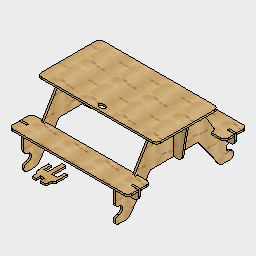
Picnic Table To Go Assembly v11 (Autodesk Fusion 360 design; units mm, degrees)
Autodesk Fusion 360 part; units mm, degrees
note: some values were not read from the file. Set by a fixed rule: which sketch regions a step uses.
sketch "Sketch1" plane through (0, 0, 0) normal (1, 0, 0) x (0, 1, 0) in component "Table Leg 1"
  line L0 (0, 0) -> (0, 304.8)
  line L1 (0, 304.8) -> (101.6, 304.8)
  line L2 (101.6, 304.8) -> (101.6, 234.95)
  line L3 (101.6, 234.95) -> (120.6183, 234.95)
  line L4 (120.6183, 234.95) -> (120.6183, 304.8)
  line L5 (120.6183, 304.8) -> (222.25, 304.8)
  line L6 (222.25, 304.8) -> (222.25, 323.8182)
  line L7 (222.25, 323.8182) -> (184.15, 323.8182)
  line L8 (184.15, 323.8182) -> (355.6, 609.6)
  line L9 (355.6, 609.6) -> (812.8, 609.6)
  line L10 (812.8, 609.6) -> (984.25, 323.8182)
  line L11 (984.25, 323.8182) -> (946.15, 323.8182)
  line L12 (946.15, 323.8182) -> (946.15, 304.8)
  line L13 (946.15, 304.8) -> (1047.7818, 304.8)
  line L14 (1047.7818, 304.8) -> (1047.7817, 234.95)
  line L15 (1047.7818, 234.95) -> (1066.8, 234.95)
  line L16 (1066.8, 234.95) -> (1066.8, 304.8)
  line L17 (1066.8, 304.8) -> (1168.4, 304.8)
  line L18 (1168.4, 304.8) -> (1168.4, 0)
  line L19 (1168.4, 0) -> (1034.5613, 0)
  line L20 (1034.5613, 0) -> (819.15, 304.8)
  line L21 (819.15, 304.8) -> (349.25, 304.8)
  line L22 (349.25, 304.8) -> (133.8387, 0)
  line L23 (133.8387, 0) -> (0, 0)
  line L24 (584.2, 304.8) -> (584.2, 609.6) construction
  line L25 (574.6909, 609.6) -> (574.6909, 635)
  line L26 (574.6909, 635) -> (574.6909, 493.776)
  line L27 (574.6909, 493.776) -> (593.7091, 493.776)
  line L28 (593.7091, 493.776) -> (593.7091, 609.6)
  circle A0 centre (482.6, 558.8) radius 50.8
  line L29 (431.8, 558.8) -> (533.4, 558.8)
  circle A1 centre (685.8, 558.8) radius 50.8
  line L30 (635, 558.8) -> (736.6, 558.8)
  arc A2 (114.1106, 0) -> (145.2246, 16.1108) centre (114.1106, 38.1) ccw
  arc A3 (38.1, 76.2) -> (38.1, 0) centre (38.1, 38.1) ccw
  arc A4 (0, 190.5) -> (38.1, 152.4) centre (38.1, 190.5) ccw
  arc A5 (38.1, 76.2) -> (38.1, 152.4) centre (38.1, 114.3) ccw
  arc A6 (368.9781, 304.8) -> (337.864, 288.6892) centre (368.9781, 266.7) ccw
  arc A7 (830.536, 288.6892) -> (799.4219, 304.8) centre (799.4219, 266.7) ccw
  arc A8 (1023.1754, 16.1108) -> (1054.2894, 0) centre (1054.2894, 38.1) ccw
  arc A9 (1130.3, 152.4) -> (1168.4, 190.5) centre (1130.3, 190.5) ccw
  arc A10 (1130.3, 152.4) -> (1130.3, 76.2) centre (1130.3, 114.3) ccw
  arc A11 (1130.3, 0) -> (1130.3, 76.2) centre (1130.3, 38.1) ccw
  arc A12 (823.8984, 591.1007) -> (791.2269, 609.6) centre (791.2269, 571.5) ccw
  arc A13 (377.1731, 609.6) -> (344.5016, 591.1007) centre (377.1731, 571.5) ccw
  arc A14 (195.6889, 343.0518) -> (206.5793, 323.8182) centre (206.5793, 336.5183) ccw
  arc A15 (961.8207, 323.8182) -> (972.7111, 343.0518) centre (961.8207, 336.5182) ccw
  line L31 (38.1, 114.3) -> (48.26, 114.3)
  line L32 (48.26, 114.3) -> (76.2, 114.3) construction
  line L33 (1130.3, 114.3) -> (1092.2, 114.3) construction
  dimension "d4" = 304.8
  dimension "d5" = 19.0183
  dimension "d6" = 38.1
  dimension "d7" = 19.0183
  dimension "d8" = 69.85
  dimension "d9" = 184.15
  dimension "d10" = 101.6
  dimension "d11" = 184.15
  dimension "d12" = 254
  dimension "d13" = 469.9
  dimension "d14" = 1168.4
  dimension "d15" = 304.8
  dimension "d16" = 374.65
  dimension "d17" = 115.824
  dimension "d18" = 19.0183
  dimension "d19" = 101.6
  dimension "d20" = 101.6
  dimension "d21" = 101.6
  dimension "d23" = 38.1
  dimension "d24" = 38.1
  dimension "d25" = 38.1
  dimension "d26" = 76.2
  dimension "d27" = 38.1
  dimension "d28" = 38.1
  dimension "d29" = 38.1
  dimension "d30" = 38.1
  dimension "d31" = 38.1
  dimension "d32" = 38.1
  dimension "d33" = 38.1
  dimension "d34" = 76.2
  dimension "d35" = 12.7
  dimension "d36" = 12.7
  dimension "d37" = 38.1
  dimension "d38" = 38.1
  dimension "d200" = 225.425
  dimension "d230" = 0
  dimension "d231" = 0
  dimension "d232" = 0
  dimension "d233" = 0
  dimension "d270" = 0
  dimension "d271" = 0
  dimension "d272" = 0
  dimension "d273" = 0
  dimension "d495" = 0
  dimension "d496" = 0
  dimension "d497" = 0
  dimension "d498" = 0
  dimension "d543" = 457.2
  dimension "d545" = 70.48
  dimension "d556" = 0
  dimension "d557" = 0
  dimension "d558" = 0
  dimension "d559" = 0
  dimension "d564" = 70.5
  dimension "d566" = 0
  dimension "d567" = 0
  dimension "d568" = 0
  dimension "d569" = 0
  dimension "d601" = 609.6
  dimension "d602" = 311.15
  dimension "d604" = 0
  dimension "d605" = 0
  dimension "d606" = 0
  dimension "d607" = 0
  dimension "d636" = 0
  dimension "d637" = 0
  dimension "d638" = 0
  dimension "d639" = 0
  dimension "d652" = 0
  dimension "d653" = 0
  dimension "d654" = 0
  dimension "d655" = 0
  measures "d4" distance of L0.start L0.end
  measures "d5" distance of L5.end L6.end
  measures "d6" distance of L6.end L7.end
  measures "d7" distance of L2.end L3.end
  measures "d8" distance of L3.end L4.end
  measures "d10" distance of L0.end L1.end
  measures "d11" distance of L0 L7.end
  measures "d13" distance of L20.end L21.end
  measures "d14" distance of L0 L18
  measures "d15" distance of L9 L21
  measures "d17" distance of L27.end L28.end
  measures "d18" distance of L26.end L27.end
  measures "d19" distance of L24 A0.centre
  measures "d20" diameter of A0
  measures "d21" distance of L24 A1.centre
  measures "d23" radius of A3
  measures "d24" radius of A5
  measures "d25" radius of A4
  measures "d26" distance of L0 L32.end
  measures "d27" radius of A2
  measures "d28" radius of A6
  measures "d29" radius of A7
  measures "d30" radius of A8
  measures "d31" radius of A11
  measures "d32" radius of A10
  measures "d33" radius of A9
  measures "d34" distance of L18 L33.end
  measures "d35" radius of A14
  measures "d36" radius of A15
  measures "d37" radius of A12
  measures "d38" radius of A13
  measures "d543" distance of L8.end L9.end
  measures "d564" angle of L20 L22
  measures "d601" distance of L8.end L23
extrude "Extrude1" add sketch "Sketch1" along normal blind 18.2563 contours A1 L30 | A0 L29 | L0 L1 L2 L3 L4 L5 L6 L7 L8 L9 L10 L11 L12 L13 L14 L15 L16 L17 L18 L19 L20 L21 L22 L23 L26 L27 L28 A2 A3 A4 A5 A8 A9 A10 A11 A12 A13 A14 A15 picked at (681.0293, 575.0474) picked at (477.8293, 575.0474) makes body 1 in component "Table Leg 1"
sketch "Sketch1 (2)" plane through (0, 0, 0) normal (1, 0, 0) x (0, 1, 0) in component "Table Leg 2"
  line L0 (0, 0) -> (0, 304.8)
  line L1 (0, 304.8) -> (101.6, 304.8)
  line L2 (101.6, 304.8) -> (101.6, 234.95)
  line L3 (101.6, 234.95) -> (120.6183, 234.95)
  line L4 (120.6183, 234.95) -> (120.6183, 304.8)
  line L5 (120.6183, 304.8) -> (222.25, 304.8)
  line L6 (222.25, 304.8) -> (222.25, 323.8182)
  line L7 (222.25, 323.8182) -> (184.15, 323.8182)
  line L8 (184.15, 323.8182) -> (355.6, 609.6)
  line L9 (355.6, 609.6) -> (812.8, 609.6)
  line L10 (812.8, 609.6) -> (984.25, 323.8182)
  line L11 (984.25, 323.8182) -> (946.15, 323.8183)
  line L12 (946.15, 323.8183) -> (946.15, 304.8)
  line L13 (946.15, 304.8) -> (1047.7818, 304.8)
  line L14 (1047.7818, 304.8) -> (1047.7817, 234.95)
  line L15 (1047.7818, 234.95) -> (1066.8, 234.95)
  line L16 (1066.8, 234.95) -> (1066.8, 304.8)
  line L17 (1066.8, 304.8) -> (1168.4, 304.8)
  line L18 (1168.4, 304.8) -> (1168.4, 0)
  line L19 (1168.4, 0) -> (1034.5613, 0)
  line L20 (1034.5613, 0) -> (819.15, 304.8)
  line L21 (819.15, 304.8) -> (349.25, 304.8)
  line L22 (349.25, 304.8) -> (133.8387, 0)
  line L23 (133.8387, 0) -> (0, 0)
  line L24 (584.2, 304.8) -> (584.2, 609.6) construction
  line L25 (574.6909, 609.6) -> (574.6909, 635)
  line L26 (574.6909, 635) -> (574.6909, 493.776)
  line L27 (574.6909, 493.776) -> (593.7091, 493.776)
  line L28 (593.7091, 493.776) -> (593.7091, 609.6)
  circle A0 centre (482.6, 558.8) radius 50.8
  line L29 (431.8, 558.8) -> (533.4, 558.8)
  circle A1 centre (685.8, 558.8) radius 50.8
  line L30 (635, 558.8) -> (736.6, 558.8)
  arc A2 (114.1106, 0) -> (145.2246, 16.1108) centre (114.1106, 38.1) ccw
  arc A3 (38.1, 76.2) -> (38.1, 0) centre (38.1, 38.1) ccw
  arc A4 (0, 190.5) -> (38.1, 152.4) centre (38.1, 190.5) ccw
  arc A5 (38.1, 76.2) -> (38.1, 152.4) centre (38.1, 114.3) ccw
  arc A6 (368.9781, 304.8) -> (337.864, 288.6892) centre (368.9781, 266.7) ccw
  arc A7 (830.536, 288.6892) -> (799.4219, 304.8) centre (799.4219, 266.7) ccw
  arc A8 (1023.1754, 16.1108) -> (1054.2894, 0) centre (1054.2894, 38.1) ccw
  arc A9 (1130.3, 152.4) -> (1168.4, 190.5) centre (1130.3, 190.5) ccw
  arc A10 (1130.3, 152.4) -> (1130.3, 76.2) centre (1130.3, 114.3) ccw
  arc A11 (1130.3, 0) -> (1130.3, 76.2) centre (1130.3, 38.1) ccw
  arc A12 (823.8984, 591.1007) -> (791.2269, 609.6) centre (791.2269, 571.5) ccw
  arc A13 (377.1731, 609.6) -> (344.5016, 591.1007) centre (377.1731, 571.5) ccw
  arc A14 (195.6889, 343.0518) -> (206.5793, 323.8182) centre (206.5793, 336.5182) ccw
  arc A15 (961.8207, 323.8182) -> (972.7111, 343.0518) centre (961.8207, 336.5182) ccw
  line L31 (38.1, 114.3) -> (48.26, 114.3)
  line L32 (48.26, 114.3) -> (76.2, 114.3) construction
  line L33 (1130.3, 114.3) -> (1092.2, 114.3) construction
  dimension "d4_1" = 304.8
  dimension "d5_1" = 19.0183
  dimension "d6_1" = 38.1
  dimension "d7_1" = 19.0183
  dimension "d8_1" = 69.85
  dimension "d9_1" = 184.15
  dimension "d10_1" = 101.6
  dimension "d11_1" = 184.15
  dimension "d12_1" = 254
  dimension "d13_1" = 469.9
  dimension "d14_1" = 1168.4
  dimension "d15_1" = 304.8
  dimension "d16_1" = 374.65
  dimension "d17_1" = 115.824
  dimension "d18_1" = 19.0183
  dimension "d19_1" = 101.6
  dimension "d20_1" = 101.6
  dimension "d21_1" = 101.6
  dimension "d23_1" = 38.1
  dimension "d24_1" = 38.1
  dimension "d25_1" = 38.1
  dimension "d26_1" = 76.2
  dimension "d27_1" = 38.1
  dimension "d28_1" = 38.1
  dimension "d29_1" = 38.1
  dimension "d30_1" = 38.1
  dimension "d31_1" = 38.1
  dimension "d32_1" = 38.1
  dimension "d33_1" = 38.1
  dimension "d34_1" = 76.2
  dimension "d35_1" = 12.7
  dimension "d36_1" = 12.7
  dimension "d37_1" = 38.1
  dimension "d38_1" = 38.1
  dimension "d218" = 0
  dimension "d219" = 0
  dimension "d220" = 0
  dimension "d221" = 0
  dimension "d254" = 0
  dimension "d255" = 0
  dimension "d256" = 0
  dimension "d257" = 0
  dimension "d262" = 0
  dimension "d263" = 0
  dimension "d264" = 0
  dimension "d265" = 0
  dimension "d471" = 0
  dimension "d472" = 0
  dimension "d473" = 0
  dimension "d474" = 0
  dimension "d487" = 0
  dimension "d488" = 0
  dimension "d489" = 0
  dimension "d490" = 0
  dimension "d544" = 457.2
  dimension "d548" = 0
  dimension "d549" = 0
  dimension "d550" = 0
  dimension "d551" = 0
  dimension "d565" = 70.5
  dimension "d603" = 609.6
  dimension "d628" = 0
  dimension "d629" = 0
  dimension "d630" = 0
  dimension "d631" = 0
  measures "d4_1" distance of L0.start L0.end
  measures "d5_1" distance of L5.end L6.end
  measures "d6_1" distance of L6.end L7.end
  measures "d7_1" distance of L2.end L3.end
  measures "d8_1" distance of L3.end L4.end
  measures "d10_1" distance of L0.end L1.end
  measures "d11_1" distance of L0 L7.end
  measures "d13_1" distance of L20.end L21.end
  measures "d14_1" distance of L0 L18
  measures "d15_1" distance of L9 L21
  measures "d17_1" distance of L27.end L28.end
  measures "d18_1" distance of L26.end L27.end
  measures "d19_1" distance of L24 A0.centre
  measures "d20_1" diameter of A0
  measures "d21_1" distance of L24 A1.centre
  measures "d23_1" radius of A3
  measures "d24_1" radius of A5
  measures "d25_1" radius of A4
  measures "d26_1" distance of L0 L32.end
  measures "d27_1" radius of A2
  measures "d28_1" radius of A6
  measures "d29_1" radius of A7
  measures "d30_1" radius of A8
  measures "d31_1" radius of A11
  measures "d32_1" radius of A10
  measures "d33_1" radius of A9
  measures "d34_1" distance of L18 L33.end
  measures "d35_1" radius of A14
  measures "d36_1" radius of A15
  measures "d37_1" radius of A12
  measures "d38_1" radius of A13
  measures "d544" distance of L8.end L9.end
  measures "d565" angle of L20 L22
  measures "d603" distance of L8.end L23
extrude "Extrude1'" add sketch "Sketch1 (2)" along normal blind 18.2563 separate body contours A1 L30 | A0 L29 | L0 L1 L2 L3 L4 L5 L6 L7 L8 L9 L10 L11 L12 L13 L14 L15 L16 L17 L18 L19 L20 L21 L22 L23 L26 L27 L28 A2 A3 A4 A5 A8 A9 A10 A11 A12 A13 A14 A15 picked at (690.3983, 577.4573) picked at (480.1901, 575.561) makes body 2 in component "Table Leg 2"
sketch "Sketch1 (3)" plane through (0, 0, 0) normal (0, 1, 0) x (1, 0, 0) in component "Tabletop Support"
  line L0 (-50.8, -304.8) -> (1117.6, -304.8)
  line L1 (1117.6, -304.8) -> (1066.8, 0)
  line L2 (1066.8, 0) -> (990.6, 0)
  line L3 (990.6, 0) -> (990.6, -188.976)
  line L4 (990.6, -188.976) -> (971.5818, -188.976)
  line L5 (971.5818, -188.976) -> (971.5818, 0)
  line L6 (971.5818, 0) -> (887.6566, 0)
  line L7 (887.6566, 0) -> (762, -177.8)
  line L8 (762, -177.8) -> (304.8, -177.8)
  line L9 (304.8, -177.8) -> (179.1434, 0)
  line L10 (179.1434, 0) -> (95.2182, 0)
  line L11 (95.2182, 0) -> (95.2183, -188.976)
  line L12 (95.2183, -188.976) -> (76.2, -188.976)
  line L13 (76.2, -188.976) -> (76.2, 0)
  line L14 (76.2, 0) -> (0, 0)
  line L15 (0, 0) -> (-50.8, -304.8)
  line L16 (533.4, -177.8) -> (533.4, -304.8) construction
  arc A0 (1072.1061, -31.8364) -> (1034.5245, 0) centre (1034.5245, -38.1) ccw
  arc A1 (907.3847, 0) -> (876.2707, -16.1108) centre (907.3847, -38.1) ccw
  arc A2 (190.5293, -16.1108) -> (159.4153, 0) centre (159.4153, -38.1) ccw
  arc A3 (32.2755, 0) -> (-5.3061, -31.8364) centre (32.2755, -38.1) ccw
  dimension "d41" = 355.6
  dimension "d42" = 19.0183
  dimension "d43" = 50.8
  dimension "d44" = 76.2
  dimension "d45" = 184.15
  dimension "d46" = 115.824
  dimension "d48" = 127
  dimension "d49" = 457.2
  dimension "d50" = 374.65
  dimension "d51" = 38.1
  dimension "d52" = 38.1
  dimension "d53" = 38.1
  dimension "d54" = 38.1
  dimension "d201" = 188.976
  dimension "d242" = 0
  dimension "d243" = 0
  dimension "d244" = 0
  dimension "d245" = 0
  dimension "d455" = 0
  dimension "d456" = 0
  dimension "d457" = 0
  dimension "d458" = 0
  dimension "d463" = 0
  dimension "d464" = 0
  dimension "d465" = 0
  dimension "d466" = 0
  dimension "d479" = 0
  dimension "d480" = 0
  dimension "d481" = 0
  dimension "d482" = 0
  dimension "d546" = 70.5
  dimension "d547" = 1168.4
  measures "d42" distance of L11.end L12.end
  measures "d43" distance of L0.start L14.end
  measures "d44" distance of L13.end L14.end
  measures "d46" distance of L0 L12
  measures "d48" distance of L0 L8
  measures "d49" distance of L7.end L8.end
  measures "d51" radius of A3
  measures "d52" radius of A2
  measures "d53" radius of A1
  measures "d54" radius of A0
  measures "d201" distance of L12 L14
  measures "d546" angle of L7 L9
  measures "d547" distance of L0.start L0.end
extrude "Extrude1''" add sketch "Sketch1 (3)" along normal blind 18.2563 separate body contours L0 L1 L2 L3 L4 L5 L6 L7 L8 L9 L10 L11 L12 L13 L14 L15 A0 A1 A2 A3 makes body 3 in component "Tabletop Support"
sketch "Sketch1 (4)" plane through (0, 0, 0) normal (0, 0, 1) x (1, 0, 0) in component "Seat 1"
  line L0 (0, 0) -> (1168.4, 0)
  line L1 (1168.4, 0) -> (1168.4, 222.25)
  line L2 (1168.4, 222.25) -> (0, 222.25)
  line L3 (0, 222.25) -> (0, 0)
  line L4 (1168.4, 120.6341) -> (1098.55, 120.6341)
  line L5 (1098.55, 120.6341) -> (1098.55, 101.6159)
  line L6 (1098.55, 101.6159) -> (1168.4, 101.6159)
  line L7 (1168.4, 101.6159) -> (1168.4, 120.6341)
  line L8 (0, 120.6341) -> (69.85, 120.6341)
  line L9 (69.85, 120.6341) -> (69.85, 101.6159)
  line L10 (69.85, 101.6159) -> (0, 101.6159)
  line L11 (0, 101.6159) -> (0, 120.6341)
  line L12 (0, 111.125) -> (1168.4, 111.125) construction
  arc A0 (38.1, 222.25) -> (0, 184.15) centre (38.1, 184.15) ccw
  arc A1 (0, 38.1) -> (38.1, 0) centre (38.1, 38.1) ccw
  arc A2 (1130.3, 0) -> (1168.4, 38.1) centre (1130.3, 38.1) ccw
  arc A3 (1168.4, 184.15) -> (1130.3, 222.25) centre (1130.3, 184.15) ccw
  dimension "d81" = 1168.4
  dimension "d82" = 222.25
  dimension "d83" = 19.0183
  dimension "d84" = 69.85
  dimension "d85" = 38.1
  dimension "d86" = 38.1
  dimension "d87" = 38.1
  dimension "d88" = 38.1
  dimension "d314" = 0
  dimension "d315" = 0
  dimension "d316" = 0
  dimension "d317" = 0
  dimension "d446" = 0
  dimension "d447" = 0
  dimension "d448" = 0
  dimension "d449" = 0
  dimension "d684" = 0
  dimension "d685" = 0
  dimension "d686" = 0
  dimension "d687" = 0
  dimension "d725" = 0
  dimension "d726" = 0
  dimension "d727" = 0
  dimension "d728" = 0
  dimension "d733" = 0
  dimension "d734" = 0
  dimension "d735" = 0
  dimension "d736" = 0
  measures "d81" distance of L1.end L2.end
  measures "d82" distance of L0.end L1.end
  measures "d83" distance of L8.end L9.end
  measures "d84" distance of L8.start L8.end
  measures "d85" radius of A1
  measures "d86" radius of A0
  measures "d87" radius of A2
  measures "d88" radius of A3
extrude "Extrude1'''" add sketch "Sketch1 (4)" along normal blind 18.2563 separate body contours L0 L1 L2 L3 L4 L5 L6 L8 L9 L10 A0 A1 A2 A3 makes body 4 in component "Seat 1"
sketch "Sketch1 (5)" plane through (0, 0, 0) normal (0, 0, 1) x (1, 0, 0) in component "Seat 2"
  line L0 (0, 0) -> (1168.4, 0)
  line L1 (1168.4, 0) -> (1168.4, 222.25)
  line L2 (1168.4, 222.25) -> (0, 222.25)
  line L3 (0, 222.25) -> (0, 0)
  line L4 (1168.4, 120.6341) -> (1098.55, 120.6341)
  line L5 (1098.55, 120.6341) -> (1098.55, 101.6159)
  line L6 (1098.55, 101.6159) -> (1168.4, 101.6159)
  line L7 (1168.4, 101.6159) -> (1168.4, 120.6341)
  line L8 (0, 120.6341) -> (69.85, 120.6341)
  line L9 (69.85, 120.6341) -> (69.85, 101.6159)
  line L10 (69.85, 101.6159) -> (0, 101.6159)
  line L11 (0, 101.6159) -> (0, 120.6341)
  line L12 (0, 111.125) -> (1168.4, 111.125) construction
  arc A0 (38.1, 222.25) -> (0, 184.15) centre (38.1, 184.15) ccw
  arc A1 (0, 38.1) -> (38.1, 0) centre (38.1, 38.1) ccw
  arc A2 (1130.3, 0) -> (1168.4, 38.1) centre (1130.3, 38.1) ccw
  arc A3 (1168.4, 184.15) -> (1130.3, 222.25) centre (1130.3, 184.15) ccw
  dimension "d81_1" = 1168.4
  dimension "d82_1" = 222.25
  dimension "d83_1" = 19.0183
  dimension "d84_1" = 69.85
  dimension "d85_1" = 38.1
  dimension "d86_1" = 38.1
  dimension "d87_1" = 38.1
  dimension "d88_1" = 38.1
  dimension "d302" = 0
  dimension "d303" = 0
  dimension "d304" = 0
  dimension "d305" = 0
  dimension "d438" = 0
  dimension "d439" = 0
  dimension "d440" = 0
  dimension "d441" = 0
  dimension "d519" = 0
  dimension "d520" = 0
  dimension "d521" = 0
  dimension "d522" = 0
  dimension "d590" = 0
  dimension "d591" = 0
  dimension "d592" = 0
  dimension "d593" = 0
  dimension "d676" = 0
  dimension "d677" = 0
  dimension "d678" = 0
  dimension "d679" = 0
  dimension "d717" = 0
  dimension "d718" = 0
  dimension "d719" = 0
  dimension "d720" = 0
  measures "d81_1" distance of L1.end L2.end
  measures "d82_1" distance of L0.end L1.end
  measures "d83_1" distance of L8.end L9.end
  measures "d84_1" distance of L8.start L8.end
  measures "d85_1" radius of A1
  measures "d86_1" radius of A0
  measures "d87_1" radius of A2
  measures "d88_1" radius of A3
extrude "Extrude1''''" add sketch "Sketch1 (5)" along normal blind 18.2563 separate body contours L0 L1 L2 L3 L4 L5 L6 L8 L9 L10 A0 A1 A2 A3 makes body 5 in component "Seat 2"
sketch "Sketch1 (6)" plane through (0, 0, 0) normal (0, 1, 0) x (1, 0, 0) in component "Seat Support 1"
  line L0 (0, 0) -> (1168.4, 0)
  line L1 (1168.4, 0) -> (1168.4, -101.6)
  line L2 (1168.4, -101.6) -> (0, -101.6)
  line L3 (0, -101.6) -> (0, 0)
  line L4 (0, -50.8) -> (1168.4, -50.8) construction
  line L5 (69.85, -101.6) -> (1098.55, -101.6)
  line L6 (1098.55, -101.6) -> (1098.55, -82.5817)
  line L7 (1098.55, -82.5817) -> (69.85, -82.5817)
  line L8 (69.85, -82.5817) -> (69.85, -101.6)
  line L9 (584.2, 0) -> (584.2, -101.6) construction
  arc A0 (38.1, 0) -> (0, -38.1) centre (38.1, -38.1) ccw
  arc A1 (1168.4, -38.1) -> (1130.3, 0) centre (1130.3, -38.1) ccw
  line L10 (127, 0) -> (146.0182, 0)
  line L11 (146.0182, 0) -> (146.0182, -12.7)
  line L12 (146.0182, -12.7) -> (127, -12.7)
  line L13 (127, -12.7) -> (127, 0)
  line L14 (1022.3818, 0) -> (1041.4, 0)
  line L15 (1041.4, 0) -> (1041.4, -12.7)
  line L16 (1041.4, -12.7) -> (1022.3818, -12.7)
  line L17 (1022.3818, -12.7) -> (1022.3818, 0)
  dimension "d91" = 1168.4
  dimension "d92" = 101.6
  dimension "d93" = 19.0183
  dimension "d94" = 69.85
  dimension "d95" = 38.1
  dimension "d96" = 38.1
  dimension "d99" = 19.0183
  dimension "d100" = 127
  dimension "d198" = 69.8818
  dimension "d290" = 0
  dimension "d291" = 0
  dimension "d292" = 0
  dimension "d293" = 0
  dimension "d422" = 0
  dimension "d423" = 0
  dimension "d424" = 0
  dimension "d425" = 0
  dimension "d503" = 0
  dimension "d504" = 0
  dimension "d505" = 0
  dimension "d506" = 0
  dimension "d574" = 0
  dimension "d575" = 0
  dimension "d576" = 0
  dimension "d577" = 0
  dimension "d660" = 0
  dimension "d661" = 0
  dimension "d662" = 0
  dimension "d663" = 0
  dimension "d701" = 0
  dimension "d702" = 0
  dimension "d703" = 0
  dimension "d704" = 0
  measures "d91" distance of L1.end L2.end
  measures "d92" distance of L0.start L2.end
  measures "d93" distance of L5.start L7.end
  measures "d94" distance of L3 L8
  measures "d95" radius of A0
  measures "d96" radius of A1
  measures "d99" distance of L11.end L12.end
  measures "d100" distance of L3 L13
  measures "d198" distance of L7 L12
extrude "Extrude1'''''" add sketch "Sketch1 (6)" along normal blind 18.2563 separate body contours L0 L1 L2 L3 L6 L7 L8 A0 A1 L11 L12 L13 L15 L16 L17 makes body 6 in component "Seat Support 1"
sketch "Sketch1 (7)" plane through (0, 0, 0) normal (0, 1, 0) x (1, 0, 0) in component "Seat Support 2"
  line L0 (0, 0) -> (1168.4, 0)
  line L1 (1168.4, 0) -> (1168.4, -101.6)
  line L2 (1168.4, -101.6) -> (0, -101.6)
  line L3 (0, -101.6) -> (0, 0)
  line L4 (0, -50.8) -> (1168.4, -50.8) construction
  line L5 (69.85, -101.6) -> (1098.55, -101.6)
  line L6 (1098.55, -101.6) -> (1098.55, -82.5817)
  line L7 (1098.55, -82.5817) -> (69.85, -82.5817)
  line L8 (69.85, -82.5817) -> (69.85, -101.6)
  line L9 (584.2, 0) -> (584.2, -101.6) construction
  arc A0 (38.1, 0) -> (0, -38.1) centre (38.1, -38.1) ccw
  arc A1 (1168.4, -38.1) -> (1130.3, 0) centre (1130.3, -38.1) ccw
  line L10 (127, 0) -> (146.0182, 0)
  line L11 (146.0182, 0) -> (146.0182, -12.7)
  line L12 (146.0182, -12.7) -> (127, -12.7)
  line L13 (127, -12.7) -> (127, 0)
  line L14 (1022.3818, 0) -> (1041.4, 0)
  line L15 (1041.4, 0) -> (1041.4, -12.7)
  line L16 (1041.4, -12.7) -> (1022.3818, -12.7)
  line L17 (1022.3818, -12.7) -> (1022.3818, 0)
  dimension "d91_1" = 1168.4
  dimension "d92_1" = 101.6
  dimension "d93_1" = 19.0183
  dimension "d94_1" = 69.85
  dimension "d95_1" = 38.1
  dimension "d96_1" = 38.1
  dimension "d99_1" = 19.0183
  dimension "d100_1" = 127
  dimension "d199" = 69.8818
  dimension "d278" = 0
  dimension "d279" = 0
  dimension "d280" = 0
  dimension "d281" = 0
  dimension "d430" = 0
  dimension "d431" = 0
  dimension "d432" = 0
  dimension "d433" = 0
  dimension "d511" = 0
  dimension "d512" = 0
  dimension "d513" = 0
  dimension "d514" = 0
  dimension "d582" = 0
  dimension "d583" = 0
  dimension "d584" = 0
  dimension "d585" = 0
  dimension "d668" = 0
  dimension "d669" = 0
  dimension "d670" = 0
  dimension "d671" = 0
  dimension "d709" = 0
  dimension "d710" = 0
  dimension "d711" = 0
  dimension "d712" = 0
  measures "d91_1" distance of L1.end L2.end
  measures "d92_1" distance of L0.start L2.end
  measures "d93_1" distance of L5.start L7.end
  measures "d94_1" distance of L3 L8
  measures "d95_1" radius of A0
  measures "d96_1" radius of A1
  measures "d99_1" distance of L11.end L12.end
  measures "d100_1" distance of L3 L13
  measures "d199" distance of L7 L12
extrude "Extrude1''''''" add sketch "Sketch1 (7)" along normal blind 18.2563 separate body contours L0 L1 L2 L3 L6 L7 L8 A0 A1 L11 L12 L13 L15 L16 L17 makes body 7 in component "Seat Support 2"
sketch "Sketch1 (8)" plane through (0, 0, 0) normal (0, 0, 1) x (1, 0, 0) in component "Tabletop"
  line L0 (0, 0) -> (1168.4, 0)
  line L1 (1168.4, 0) -> (1168.4, 609.6)
  line L2 (1168.4, 609.6) -> (0, 609.6)
  line L3 (0, 609.6) -> (0, 0)
  arc A0 (0, 38.1) -> (38.1, 0) centre (38.1, 38.1) ccw
  arc A1 (38.1, 609.6) -> (0, 571.5) centre (38.1, 571.5) ccw
  arc A2 (1168.4, 571.5) -> (1130.3, 609.6) centre (1130.3, 571.5) ccw
  arc A3 (1130.3, 0) -> (1168.4, 38.1) centre (1130.3, 38.1) ccw
  arc A4 (620.121, 50.8) -> (548.279, 50.8) centre (584.2, 38.1) ccw
  arc A5 (548.279, 50.8) -> (620.121, 50.8) centre (584.2, 63.5) ccw
  line L4 (584.2, 0) -> (584.2, 609.6) construction
  line L5 (584.2, 25.4) -> (584.2, 76.2) construction
  dimension "d150" = 38.1
  dimension "d151" = 38.1
  dimension "d152" = 38.1
  dimension "d153" = 38.1
  dimension "d154" = 609.6
  dimension "d155" = 1168.4
  dimension "d156" = 38.1
  dimension "d157" = 38.1
  dimension "d159" = 25.4
  dimension "d160" = 76.2
  dimension "d206" = 0
  dimension "d207" = 0
  dimension "d208" = 0
  dimension "d209" = 0
  measures "d150" radius of A0
  measures "d151" radius of A1
  measures "d152" radius of A3
  measures "d153" radius of A2
  measures "d154" distance of L0.start L2.end
  measures "d155" distance of L0.start L0.end
  measures "d156" radius of A5
  measures "d157" radius of A4
  measures "d159" distance of L0 L5.start
  measures "d160" distance of L0 L5.end
extrude "Extrude1'''''''" add sketch "Sketch1 (8)" along normal blind 18.2563 separate body contours L0 L1 L2 L3 A0 A1 A2 A3 makes body 8 in component "Tabletop"
sketch "Sketch2" plane through (0, 0, 0) normal (0, 0, -1) x (1, 0, 0) in component "Tabletop"
  arc A0 (620.121, -50.8) -> (548.279, -50.8) centre (584.2, -63.5) ccw
  arc A1 (548.279, -50.8) -> (620.121, -50.8) centre (584.2, -38.1) ccw
  arc A2 (1168.4, -38.1) -> (1130.3, 0) centre (1130.3, -38.1) ccw
  line L0 (1130.3, 0) -> (38.1, 0)
  arc A3 (38.1, 0) -> (0, -38.1) centre (38.1, -38.1) ccw
  line L1 (0, -38.1) -> (0, -571.5)
  arc A4 (0, -571.5) -> (38.1, -609.6) centre (38.1, -571.5) ccw
  line L2 (38.1, -609.6) -> (1130.3, -609.6)
  arc A5 (1130.3, -609.6) -> (1168.4, -571.5) centre (1130.3, -571.5) ccw
  line L3 (1168.4, -571.5) -> (1168.4, -38.1)
  line L4 (0, -304.8) -> (1168.4, -304.8) construction
  line L5 (145.6373, -295.2909) -> (444.0873, -295.2909)
  line L6 (444.0873, -295.2909) -> (444.0873, -230.7749)
  line L7 (444.0873, -230.7749) -> (145.6373, -230.7749)
  line L8 (145.6373, -230.7749) -> (145.6373, -295.2909)
  line L9 (145.6373, -314.3091) -> (444.0873, -314.3091)
  line L10 (444.0873, -314.3091) -> (444.0873, -378.8251)
  line L11 (444.0873, -378.8251) -> (145.6373, -378.8251)
  line L12 (145.6373, -378.8251) -> (145.6373, -314.3091)
  line L13 (1022.7628, -314.3091) -> (724.3128, -314.3091)
  line L14 (724.3128, -314.3091) -> (724.3128, -378.8251)
  line L15 (724.3128, -378.8251) -> (1022.7628, -378.8251)
  line L16 (1022.7628, -378.8251) -> (1022.7628, -314.3091)
  line L17 (1022.7628, -230.7749) -> (724.3128, -230.7749)
  line L18 (724.3128, -230.7749) -> (724.3128, -295.2909)
  line L19 (724.3128, -295.2909) -> (1022.7628, -295.2909)
  line L20 (1022.7628, -295.2909) -> (1022.7628, -230.7749)
  line L21 (444.0873, -295.2909) -> (444.0873, -314.3091) construction
  line L22 (724.3128, -295.2909) -> (724.3128, -314.3091) construction
  line L23 (145.6373, -295.2909) -> (145.6373, -97.7731)
  line L24 (1022.7628, -97.7731) -> (1022.7628, -295.2909)
  dimension "d163" = 19.0183
  dimension "d164" = 64.516
  dimension "d165" = 298.45
  measures "d163" distance of L5 L9
  measures "d164" distance of L5.start L7.end
  measures "d165" distance of L6.end L7.end
extrude "Extrude2" add sketch "Sketch2" along normal blind 18.2563 separate body contours L5 L6 L7 L8 L23 | L9 L10 L11 L12 | L13 L14 L15 L16 | L17 L18 L19 L20 L24 makes body 9 at (245.1206, 335.8145, 0) makes body 10 at (923.2794, 357.3198, 0) makes body 11 at (245.1206, 252.2802, 0) makes body 12 at (923.2794, 252.2802, 0) in component "Tabletop"
copy_body "Body->Comp1" bodies 9 removing the originals makes body 13 in component "Component"
copy_body "Body->Comp2" bodies 11 removing the originals makes body 14 in component "Component'"
copy_body "Body->Comp3" bodies 10 removing the originals makes body 15 in component "Component''"
copy_body "Body->Comp4" bodies 12 removing the originals makes body 16 in component "Component'''"
sketch "Sketch1 (9)" plane through (0, 0, 0) normal (0, 0, 1) x (1, 0, 0) in component "Carrying Clips"
  line L0 (25.4, 0) -> (63.5, 0)
  line L1 (63.5, 0) -> (63.5, 44.45)
  line L2 (63.5, 44.45) -> (101.6, 44.45)
  line L3 (101.6, 44.45) -> (101.6, 0)
  line L4 (101.6, 0) -> (158.75, 0)
  line L5 (184.15, 82.55) -> (184.15, 184.15)
  line L6 (184.15, 184.15) -> (158.75, 184.15)
  line L7 (158.75, 184.15) -> (158.75, 114.3)
  line L8 (158.75, 114.3) -> (101.6, 114.3)
  line L9 (101.6, 114.3) -> (101.6, 254)
  line L10 (101.6, 254) -> (63.5, 254)
  line L11 (63.5, 254) -> (63.5, 114.3)
  line L12 (63.5, 114.3) -> (25.4, 114.3)
  line L13 (25.4, 114.3) -> (25.4, 184.15)
  line L14 (25.4, 184.15) -> (0, 184.15)
  line L15 (0, 184.15) -> (0, 82.55)
  line L16 (0, 82.55) -> (0, 0) construction
  line L17 (0, 0) -> (25.4, 0) construction
  line L18 (25.4, 0) -> (25.4, 25.7539)
  arc A0 (0, 82.55) -> (12.7, 54.1519) centre (38.1, 82.55) ccw
  arc A1 (25.4, 25.7539) -> (12.7, 54.1519) centre (-12.7, 25.7539) ccw
  line L19 (158.75, 0) -> (158.75, 25.7539)
  arc A2 (171.45, 54.1519) -> (158.75, 25.7539) centre (196.85, 25.7539) ccw
  arc A3 (171.45, 54.1519) -> (184.15, 82.55) centre (146.05, 82.55) ccw
  line L20 (184.15, 82.55) -> (0, 82.55) construction
  dimension "d180" = 38.1
  dimension "d181" = 57.15
  dimension "d182" = 82.55
  dimension "d183" = 38.1
  dimension "d184" = 63.5
  dimension "d185" = 82.55
  dimension "d186" = 254
  dimension "d187" = 184.15
  dimension "d188" = 114.3
  dimension "d189" = 25.4
  dimension "d190" = 44.45
  dimension "d191" = 38.1
  dimension "d192" = 38.1
  dimension "d193" = 38.1
  dimension "d194" = 38.1
  dimension "d195" = 38.1
  dimension "d326" = 0
  dimension "d327" = 0
  dimension "d328" = 0
  dimension "d329" = 0
  dimension "d338" = 0
  dimension "d339" = 0
  dimension "d340" = 0
  dimension "d341" = 0
  dimension "d350" = 0
  dimension "d351" = 0
  dimension "d352" = 0
  dimension "d353" = 0
  dimension "d358" = 0
  dimension "d359" = 0
  dimension "d360" = 0
  dimension "d361" = 0
  dimension "d366" = 0
  dimension "d367" = 0
  dimension "d368" = 0
  dimension "d369" = 0
  dimension "d527" = 0
  dimension "d528" = 0
  dimension "d529" = 0
  dimension "d530" = 0
  dimension "d535" = 0
  dimension "d536" = 0
  dimension "d537" = 0
  dimension "d538" = 0
  dimension "d773" = 0
  dimension "d774" = 0
  dimension "d775" = 0
  dimension "d776" = 0
  dimension "d813" = 0
  dimension "d814" = 0
  dimension "d815" = 0
  dimension "d816" = 0
  measures "d180" distance of L11.end L12.end
  measures "d181" distance of L7.end L8.end
  measures "d182" distance of L3 L5
  measures "d183" distance of L1.end L2.end
  measures "d184" distance of L1 L15
  measures "d185" distance of L0 L15.end
  measures "d186" distance of L4 L10
  measures "d187" distance of L4 L6
  measures "d188" distance of L0 L12
  measures "d189" distance of L5.end L6.end
  measures "d190" distance of L2.end L3.end
  measures "d191" radius of A1
  measures "d192" radius of A0
  measures "d193" distance of L0.start L0.end
  measures "d194" radius of A2
  measures "d195" radius of A3
extrude "Extrude1''''''''" add sketch "Sketch1 (9)" along normal blind 18.2563 separate body makes body 17 in component "Carrying Clips"
sketch "Sketch1 (10)" plane through (0, 0, 0) normal (0, 0, 1) x (1, 0, 0) in component "Stock"
  line L0 (0, 0) -> (2438.4, 0)
  line L1 (2438.4, 0) -> (2438.4, 1219.2)
  line L2 (2438.4, 1219.2) -> (0, 1219.2)
  line L3 (0, 1219.2) -> (0, 0)
  dimension "d202" = 2438.4
  dimension "d203" = 1219.2
  dimension "d210" = 0
  dimension "d211" = 0
  dimension "d212" = 0
  dimension "d213" = 0
  dimension "d222" = 0
  dimension "d223" = 0
  dimension "d224" = 0
  dimension "d225" = 0
  dimension "d234" = 0
  dimension "d235" = 0
  dimension "d236" = 0
  dimension "d237" = 0
  dimension "d246" = 0
  dimension "d247" = 0
  dimension "d248" = 0
  dimension "d249" = 0
  dimension "d258" = 0
  dimension "d259" = 0
  dimension "d260" = 0
  dimension "d261" = 0
  dimension "d266" = 0
  dimension "d267" = 0
  dimension "d268" = 0
  dimension "d269" = 0
  dimension "d274" = 0
  dimension "d275" = 0
  dimension "d276" = 0
  dimension "d277" = 0
  dimension "d282" = 0
  dimension "d283" = 0
  dimension "d284" = 0
  dimension "d285" = 0
  dimension "d294" = 0
  dimension "d295" = 0
  dimension "d296" = 0
  dimension "d297" = 0
  dimension "d306" = 0
  dimension "d307" = 0
  dimension "d308" = 0
  dimension "d309" = 0
  dimension "d318" = 0
  dimension "d319" = 0
  dimension "d320" = 0
  dimension "d321" = 0
  dimension "d330" = 0
  dimension "d331" = 0
  dimension "d332" = 0
  dimension "d333" = 0
  dimension "d342" = 0
  dimension "d343" = 0
  dimension "d344" = 0
  dimension "d345" = 0
  dimension "d354" = 0
  dimension "d355" = 0
  dimension "d356" = 0
  dimension "d357" = 0
  dimension "d362" = 0
  dimension "d363" = 0
  dimension "d364" = 0
  dimension "d365" = 0
  dimension "d370" = 0
  dimension "d371" = 0
  dimension "d372" = 0
  dimension "d373" = 0
  dimension "d378" = 0
  dimension "d379" = 0
  dimension "d380" = 0
  dimension "d381" = 0
  dimension "d390" = 0
  dimension "d391" = 0
  dimension "d392" = 0
  dimension "d393" = 0
  dimension "d402" = 0
  dimension "d403" = 0
  dimension "d404" = 0
  dimension "d405" = 0
  dimension "d414" = 0
  dimension "d415" = 0
  dimension "d416" = 0
  dimension "d417" = 0
  dimension "d426" = 0
  dimension "d427" = 0
  dimension "d428" = 0
  dimension "d429" = 0
  dimension "d434" = 0
  dimension "d435" = 0
  dimension "d436" = 0
  dimension "d437" = 0
  dimension "d442" = 0
  dimension "d443" = 0
  dimension "d444" = 0
  dimension "d445" = 0
  dimension "d450" = 0
  dimension "d451" = 0
  dimension "d452" = 0
  dimension "d453" = 0
  dimension "d459" = 0
  dimension "d460" = 0
  dimension "d461" = 0
  dimension "d462" = 0
  dimension "d467" = 0
  dimension "d468" = 0
  dimension "d469" = 0
  dimension "d470" = 0
  dimension "d475" = 0
  dimension "d476" = 0
  dimension "d477" = 0
  dimension "d478" = 0
  dimension "d483" = 0
  dimension "d484" = 0
  dimension "d485" = 0
  dimension "d486" = 0
  dimension "d491" = 0
  dimension "d492" = 0
  dimension "d493" = 0
  dimension "d494" = 0
  dimension "d499" = 0
  dimension "d500" = 0
  dimension "d501" = 0
  dimension "d502" = 0
  dimension "d507" = 0
  dimension "d508" = 0
  dimension "d509" = 0
  dimension "d510" = 0
  dimension "d515" = 0
  dimension "d516" = 0
  dimension "d517" = 0
  dimension "d518" = 0
  dimension "d523" = 0
  dimension "d524" = 0
  dimension "d525" = 0
  dimension "d526" = 0
  dimension "d531" = 0
  dimension "d532" = 0
  dimension "d533" = 0
  dimension "d534" = 0
  dimension "d539" = 0
  dimension "d540" = 0
  dimension "d541" = 0
  dimension "d542" = 0
  dimension "d552" = 0
  dimension "d553" = 0
  dimension "d554" = 0
  dimension "d555" = 0
  dimension "d560" = 0
  dimension "d561" = 0
  dimension "d562" = 0
  dimension "d563" = 0
  dimension "d570" = 0
  dimension "d571" = 0
  dimension "d572" = 0
  dimension "d573" = 0
  dimension "d578" = 0
  dimension "d579" = 0
  dimension "d580" = 0
  dimension "d581" = 0
  dimension "d586" = 0
  dimension "d587" = 0
  dimension "d588" = 0
  dimension "d589" = 0
  dimension "d594" = 0
  dimension "d595" = 0
  dimension "d596" = 0
  dimension "d597" = 0
  dimension "d608" = 0
  dimension "d609" = 0
  dimension "d610" = 0
  dimension "d611" = 0
  dimension "d632" = 0
  dimension "d633" = 0
  dimension "d634" = 0
  dimension "d635" = 0
  dimension "d640" = 0
  dimension "d641" = 0
  dimension "d642" = 0
  dimension "d643" = 0
  dimension "d656" = 0
  dimension "d657" = 0
  dimension "d658" = 0
  dimension "d659" = 0
  dimension "d664" = 0
  dimension "d665" = 0
  dimension "d666" = 0
  dimension "d667" = 0
  dimension "d672" = 0
  dimension "d673" = 0
  dimension "d674" = 0
  dimension "d675" = 0
  dimension "d680" = 0
  dimension "d681" = 0
  dimension "d682" = 0
  dimension "d683" = 0
  dimension "d688" = 0
  dimension "d689" = 0
  dimension "d690" = 0
  dimension "d691" = 0
  dimension "d705" = 0
  dimension "d706" = 0
  dimension "d707" = 0
  dimension "d708" = 0
  dimension "d713" = 0
  dimension "d714" = 0
  dimension "d715" = 0
  dimension "d716" = 0
  dimension "d721" = 0
  dimension "d722" = 0
  dimension "d723" = 0
  dimension "d724" = 0
  dimension "d729" = 0
  dimension "d730" = 0
  dimension "d731" = 0
  dimension "d732" = 0
  dimension "d737" = 0
  dimension "d738" = 0
  dimension "d739" = 0
  dimension "d740" = 0
  dimension "d777" = 0
  dimension "d778" = 0
  dimension "d779" = 0
  dimension "d780" = 0
  dimension "d785" = 0
  dimension "d786" = 0
  dimension "d787" = 0
  dimension "d788" = 0
  dimension "d793" = 0
  dimension "d794" = 0
  dimension "d795" = 0
  dimension "d796" = 0
  dimension "d801" = 0
  dimension "d802" = 0
  dimension "d803" = 0
  dimension "d804" = 0
  dimension "d809" = 0
  dimension "d810" = 0
  dimension "d811" = 0
  dimension "d812" = 0
  dimension "d817" = 0
  dimension "d818" = 0
  dimension "d819" = 0
  dimension "d820" = 0
  dimension "d833" = 0
  dimension "d834" = 0
  dimension "d835" = 0
  dimension "d836" = 0
  dimension "d841" = 0
  dimension "d842" = 0
  dimension "d843" = 0
  dimension "d844" = 0
  dimension "d849" = 0
  dimension "d850" = 0
  dimension "d851" = 0
  dimension "d852" = 0
  dimension "d857" = 0
  dimension "d858" = 0
  dimension "d859" = 0
  dimension "d860" = 0
  measures "d202" distance of L0.start L0.end
  measures "d203" distance of L0.start L2.end
extrude "Extrude1'''''''''" add sketch "Sketch1 (10)" along normal blind 18.2563 separate body makes body 18 in component "Stock"
ref_plane "WorkPlane4" through (0, 0, 0) normal (0, 0, 1) x (1, 0, 0)
sketch "Dogbone" plane through (0, 0, 0) normal (0, 0, 1) x (1, 0, 0)
  circle A0 centre (753.0691, 154.6451) radius 3.175
  circle A1 centre (753.0691, 169.1732) radius 3.175
  circle A2 centre (753.0691, 1050.0268) radius 3.175
  circle A3 centre (753.0691, 1064.5549) radius 3.175
  circle A4 centre (1062.7268, 245.4049) radius 3.175
  circle A5 centre (1077.2549, 245.4049) radius 3.175
  circle A6 centre (1147.1049, 143.7732) radius 3.175
  circle A7 centre (1147.1049, 129.2451) radius 3.175
  circle A8 centre (1147.1049, 1089.9549) radius 3.175
  circle A9 centre (1147.1049, 1075.4268) radius 3.175
  circle A10 centre (1077.2549, 973.7951) radius 3.175
  circle A11 centre (1062.7268, 973.7951) radius 3.175
  circle A12 centre (888.2789, 616.8641) radius 3.175
  circle A13 centre (888.2789, 602.3359) radius 3.175
  circle A14 centre (1380.2268, 245.4049) radius 3.175
  circle A15 centre (1394.7549, 245.4049) radius 3.175
  circle A16 centre (1464.6049, 143.7732) radius 3.175
  circle A17 centre (1464.6049, 129.2451) radius 3.175
  circle A18 centre (1464.6049, 1089.9549) radius 3.175
  circle A19 centre (1464.6049, 1075.4268) radius 3.175
  circle A20 centre (1394.7549, 973.7951) radius 3.175
  circle A21 centre (1380.2268, 973.7951) radius 3.175
  circle A22 centre (1205.7789, 616.8641) radius 3.175
  circle A23 centre (1205.7789, 602.3359) radius 3.175
  circle A24 centre (1585.2549, 748.3701) radius 3.175
  circle A25 centre (1585.2549, 781.9799) radius 3.175
  circle A26 centre (1585.2549, 824.5701) radius 3.175
  circle A27 centre (1585.2549, 877.2299) radius 3.175
  circle A28 centre (1659.5951, 820.0799) radius 3.175
  circle A29 centre (1659.5951, 786.4701) radius 3.175
  circle A30 centre (1799.3268, 97.4951) radius 3.175
  circle A31 centre (1799.3268, 1121.7049) radius 3.175
  circle A32 centre (1724.9549, 1064.5549) radius 3.175
  circle A33 centre (1724.9549, 1050.0268) radius 3.175
  circle A34 centre (1724.9549, 169.1732) radius 3.175
  circle A35 centre (1724.9549, 154.6451) radius 3.175
  circle A36 centre (1913.6268, 97.4951) radius 3.175
  circle A37 centre (1913.6268, 1121.7049) radius 3.175
  circle A38 centre (1839.2549, 1064.5549) radius 3.175
  circle A39 centre (1839.2549, 1050.0268) radius 3.175
  circle A40 centre (1839.2549, 169.1732) radius 3.175
  circle A41 centre (1839.2549, 154.6451) radius 3.175
  circle A42 centre (2050.1359, 1126.1951) radius 3.175
  circle A43 centre (2064.6641, 1126.1951) radius 3.175
  circle A44 centre (2064.6641, 93.0049) radius 3.175
  circle A45 centre (2050.1359, 93.0049) radius 3.175
  circle A46 centre (2291.4359, 1126.1951) radius 3.175
  circle A47 centre (2305.9641, 1126.1951) radius 3.175
  circle A48 centre (2305.9641, 93.0049) radius 3.175
  circle A49 centre (2291.4359, 93.0049) radius 3.175
extrude "Extrude4" [suppressed] in component "Table Leg 1"
component "Table Leg 1" placed x (1, 0, 0) y (0, 1, 0) z (0, 0, 1) at (0, 0, 0)
component "Table Leg 2" placed x (1, 0, 0) y (0, 1, 0) z (0, 0, 1) at (895.3818, 0, 0)
component "Tabletop Support" placed x (1, 0, 0) y (0, 1, 0) z (0, 0, 1) at (-76.581, 575.0719, 304.8)
component "Seat 1" placed x (1, 0, 0) y (0, 1, 0) z (0, 0, 1) at (-127.381, -0.0159, 304.8318)
component "Seat 2" placed x (1, 0, 0) y (0, 1, 0) z (0, 0, 1) at (-127.381, 946.1659, 304.8318)
component "Seat Support 1" placed x (1, 0, 0) y (0, 1, 0) z (0, 0, 1) at (-127.381, 101.981, 222.25)
component "Seat Support 2" placed x (1, 0, 0) y (0, 1, 0) z (0, 0, 1) at (-127.381, 1048.1628, 222.25)
component "Tabletop" placed x (1, 0, 0) y (0, 1, 0) z (0, 0, 1) at (-127.381, 279.4, 609.6)
component "Carrying Clips" placed x (1, 0, 0) y (0, 1, 0) z (0, 0, 1) at (76.2, 0, 0)
component "Stock" placed x (1, 0, 0) y (0, 1, 0) z (0, 0, 1) at (0, 0, 0)
component "Carrying Clips" placed x (1, 0, 0) y (0, 1, 0) z (0, 0, 1) at (304.8, 0, 0)
component "Component" placed x (1, 0, 0) y (0, 1, 0) z (0, 0, 1) at (0, 0, 0) in component "Tabletop"
component "Component'" placed x (1, 0, 0) y (0, 1, 0) z (0, 0, 1) at (0, 0, 0) in component "Tabletop"
component "Component''" placed x (1, 0, 0) y (0, 1, 0) z (0, 0, 1) at (0, 0, 0) in component "Tabletop"
component "Component'''" placed x (1, 0, 0) y (0, 1, 0) z (0, 0, 1) at (0, 0, 0) in component "Tabletop"
equation "Ply = 0.71875 in" comment "Thickness of Plywood."
equation "Cutter = 0.25 in" comment "Diameter of cutter."
equation "Gap = 0.03 in" comment "Tolerance gap"
equation "d4 = TableH / 2"
equation "d5 = Ply + Gap"
equation "d7 = d5"
equation "d12 = TableH / 2 - 2 in"
equation "d14 = TableL"
equation "d15 = SuptD"
equation "d17 = SuptD * 0.38"
equation "d18 = d5"
equation "d21 = d19"
equation "Can = 3 in" comment "Diameter of Can"
equation "d23 = Can / 2"
equation "d24 = Can / 2"
equation "d25 = Can / 2"
equation "d27 = Can / 2"
equation "d28 = d23"
equation "d29 = d23"
equation "d30 = d23"
equation "d31 = d23"
equation "d32 = d23"
equation "d33 = d23"
equation "d34 = d26"
equation "d36 = d35"
equation "d37 = d23"
equation "d38 = d23"
equation "d39 = Ply"
equation "d4_1 = TableH / 2"
equation "d5_1 = Ply + Gap"
equation "d7_1 = d5_1"
equation "d12_1 = TableH / 2 - 2 in"
equation "d14_1 = TableL"
equation "d15_1 = SuptD"
equation "d17_1 = SuptD * 0.38"
equation "d18_1 = d5_1"
equation "d21_1 = d19_1"
equation "d23_1 = Can / 2"
equation "d24_1 = Can / 2"
equation "d25_1 = Can / 2"
equation "d27_1 = Can / 2"
equation "d28_1 = d23_1"
equation "d29_1 = d23_1"
equation "d30_1 = d23_1"
equation "d31_1 = d23_1"
equation "d32_1 = d23_1"
equation "d33_1 = d23_1"
equation "d34_1 = d26_1"
equation "d36_1 = d35_1"
equation "d37_1 = d23_1"
equation "d38_1 = d23_1"
equation "d39_1 = Ply"
equation "d42 = Ply + Gap"
equation "d46 = SuptD * 0.38"
equation "d51 = Can / 2"
equation "d52 = d51"
equation "d53 = d51"
equation "d54 = d51"
equation "d55 = Ply"
equation "d81 = TableL"
equation "d83 = Ply + Gap"
equation "d85 = d23"
equation "d86 = d23"
equation "d87 = d23"
equation "d88 = d23"
equation "d89 = Ply"
equation "d81_1 = TableL"
equation "d83_1 = Ply + Gap"
equation "d85_1 = d23"
equation "d86_1 = d23"
equation "d87_1 = d23"
equation "d88_1 = d23"
equation "d89_1 = Ply"
equation "d91 = TableL"
equation "d93 = Ply + Gap"
equation "d95 = d23"
equation "d96 = d23"
equation "d97 = Ply"
equation "d99 = Ply + Gap"
equation "d91_1 = TableL"
equation "d93_1 = Ply + Gap"
equation "d95_1 = d23"
equation "d96_1 = d23"
equation "d97_1 = Ply"
equation "d99_1 = Ply + Gap"
equation "d150 = d23"
equation "d151 = d23"
equation "d152 = d23"
equation "d153 = d23"
equation "d154 = TableW"
equation "d155 = TableL"
equation "d156 = d23"
equation "d157 = d23"
equation "d161 = Ply"
equation "d163 = Ply + Gap"
equation "d166 = Ply"
equation "d191 = d23"
equation "d192 = d23"
equation "d194 = d23"
equation "d195 = d23"
equation "d196 = Ply"
equation "d198 = d92 - d93 - 0.5 in"
equation "d199 = d198"
equation "d201 = SuptD * 0.62"
equation "d204 = Ply"
equation "d547 = TableL"
equation "TableW = 24 in" comment "Width of table"
equation "TableL = 46 in" comment "Length of table"
equation "TableH = 24 in" comment "Height of table."
equation "d601 = TableH"
equation "d603 = TableH"
equation "SuptD = 12 in" comment "Depth of Support"
